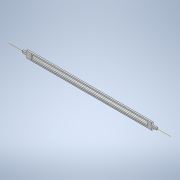
# Autodesk Inventor part: rod_3
Saved by Autodesk Inventor 2022 (Build 260153000, 153)
## iProperties
Created: 2023-04-13
Part Number: rod_3
Material: 一般
Document SubType Name: Modeling
Designer: Johnny Jou
Density: 1 g/cm^3
Appearance: 預設
Author: Johnny Jou
Autodesk Inventor part; units mm, degrees
ref_plane "YZ Plane" through (0, 0, 0) normal (1, 0, 0) x (0, 1, 0)
ref_plane "XY Plane" through (0, 0, 0) normal (0, 0, 1) x (1, 0, 0)
sketch "草圖1" plane through (0, 0, 0) normal (0, 0, 1) x (1, 0, 0)
  line L0 (0, 6) -> (0, -6)
  line L1 (0, -6) -> (-139, -6)
  line L2 (-139, -6) -> (-139, 6)
  line L3 (-149, 2) -> (-139, 2)
  line L4 (-139, 2) -> (-139, -2)
  line L5 (-139, -2) -> (-149, -2)
  line L6 (-149, -2) -> (-149, 2)
  line L7 (0, -9.6) -> (0, 15.6)
  line L8 (-148, -2) -> (-139, -2)
  line L9 (-139, -2) -> (-139, -6)
  line L10 (-139, 6) -> (-139, 2)
  line L11 (-139, 2) -> (-148, 2)
  line L12 (-139, 6) -> (0, 6)
  line L13 (139, -6) -> (139, 6)
  line L14 (139, 6) -> (139, 2)
  line L15 (139, -2) -> (139, -6)
  line L16 (139, 2) -> (148, 2)
  line L17 (149, 2) -> (139, 2)
  line L18 (148, -2) -> (139, -2)
  line L19 (139, -2) -> (149, -2)
  line L20 (149, -2) -> (149, 2)
  line L21 (139, 2) -> (139, -2)
  line L22 (0, -6) -> (139, -6)
  line L23 (139, 6) -> (0, 6)
  point P0 (0, 0)
  point P1 (0, 0)
  point P2 (0, 0)
  dimension "d0" = 10
  dimension "d1" = 139
  dimension "d2" = 4
  constraints: 48 end point, 12 symmetric about line, 3 parallel, 2 horizontal, 2 point on line, 1 coincident, 1 collinear, 1 midpoint, 1 perpendicular
  measures "d0" distance between parallel lines of L6 L2
  measures "d1" distance of L2.end L0.start
  measures "d2" distance between parallel lines of L5 L3
extrude "擠出1" add sketch "草圖1" along normal blind 3
ref_plane "工作平面1" through (0, 0, 1.5) normal (0, 0, -1) x (-1, 0, 0)
sketch "草圖2" plane through (0, 0, 3) normal (0, 0, 1) x (1, 0, 0)
  line L0 (-139, 7.5) -> (139, 7.5)
  line L1 (139, 7.5) -> (139, -7.5)
  line L2 (139, -7.5) -> (-139, -7.5)
  line L3 (-139, -7.5) -> (-139, 7.5)
  line L4 (-139, -2) -> (-139, -6) projected
  line L5 (139, -6) -> (139, -2) projected
  line L6 (139, 6) -> (-139, 6) projected
  line L7 (-129, 4.5) -> (129, 4.5)
  line L8 (129, 4.5) -> (129, -4.5)
  line L9 (129, -4.5) -> (-129, -4.5)
  line L10 (-129, -4.5) -> (-129, 4.5)
  point P0 (0, 0)
  dimension "d6" = 15
  dimension "d7" = 1.5
  dimension "d8" = 9
  dimension "d9" = 10
  dimension "d10" = 10
  dimension "d11" = 3
  constraints: 16 end point, 4 parallel, 2 collinear, 2 horizontal, 2 perpendicular
  measures "d6" distance of L2.end L0.start
  measures "d7" distance between parallel lines of L6 L0
  measures "d8" distance of L7.end L8.end
  measures "d9" distance between parallel lines of L1 L8
  measures "d10" distance between parallel lines of L3 L10
  measures "d11" distance between parallel lines of L0 L7
extrude "擠出2" add sketch "草圖2" against normal up to surface (3 mm away)
extrude "擠出3" cut sketch "草圖2" against normal up to surface (3 mm away) contours L7 L8 L9 L10
